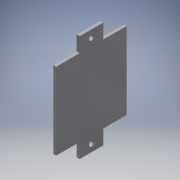
# Autodesk Inventor part: Backing Plate
Saved by Autodesk Inventor 2019 (Build 230136000, 136)
## iProperties
Created: 2020-02-21
Part Number: Backing Plate
Material: Generic
Document SubType Name: Modeling
Designer: ntb11189
Density: 1 g/cm^3
Appearance: Steel
Author: ntb11189
Autodesk Inventor part; units mm, degrees
ref_plane "YZ Plane" through (0, 0, 0) normal (1, 0, 0) x (0, 1, 0)
ref_plane "XZ Plane" through (0, 0, 0) normal (0, 1, 0) x (-1, 0, 0)
ref_plane "XY Plane" through (0, 0, 0) normal (0, 0, 1) x (1, 0, 0)
sketch "Sketch1" plane through (0, 0, 0) normal (1, 0, 0) x (0, 1, 0)
  line L0 (-181, 0) -> (-181, -40)
  line L1 (0, -40) -> (0, 0)
  line L2 (-156, -40) -> (-156, -80)
  line L3 (-156, -80) -> (-25, -80)
  line L4 (-25, -80) -> (-25, -40)
  line L5 (-156, 0) -> (-156, 40)
  line L6 (-156, 40) -> (-25, 40)
  line L7 (-25, 40) -> (-25, 0)
  line L8 (0, 0) -> (-25, 0)
  line L9 (-156, 0) -> (-181, 0)
  line L10 (-181, -40) -> (-156, -40)
  line L11 (-25, -40) -> (0, -40)
  circle A0 centre (-12.5, -20) radius 4.25
  circle A1 centre (-168.5, -20) radius 4.25
  dimension "d8" = 90
  dimension "d9" = 25
  dimension "d10" = 156
  dimension "d11" = 181
  dimension "d12" = 40
  dimension "d13" = 40
  dimension "d14" = 80
  dimension "d15" = 0
  dimension "d16" = 40
  dimension "d17" = 131
  dimension "d18" = 25
  dimension "d21" = 4.25
  dimension "d22" = 20
  dimension "d23" = 12.5
  dimension "d24" = 4.25
  dimension "d25" = 20
  dimension "d26" = 12.5
  constraints: 24 end point, 10 parallel, 2 centre point, 2 horizontal, 2 perpendicular
  measures "d8" angle of L7 L8
  measures "d9" distance between parallel lines of L1 L4
  measures "d10" distance between parallel lines of L1 L2
  measures "d11" distance between parallel lines of L1 L0
  measures "d12" distance between parallel lines of L11 L8
  measures "d13" distance between parallel lines of L6 L8
  measures "d14" distance between parallel lines of L3 L8
  measures "d15" distance between parallel lines of L9 L8
  measures "d16" distance between parallel lines of L10 L8
  measures "d17" distance between parallel lines of L5 L7
  measures "d18" distance from line of L1.end L7
  measures "d21" radius of A0
  measures "d22" distance from line of L11 A0.centre
  measures "d23" distance from line of L1 A0.centre
  measures "d24" radius of A1
  measures "d25" distance from line of L10 A1.centre
  measures "d26" distance from line of L0 A1.centre
extrude "Extrusion2" add sketch "Sketch1" along normal blind 4.8
body "Solid2"
